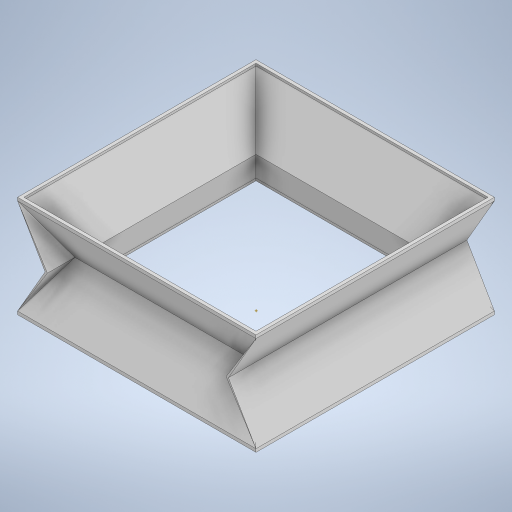
# Autodesk Inventor part: 사각형 OV-PAM 5패턴 층 한개
Saved by Autodesk Inventor 2024 (Build 280153000, 153)
## iProperties
Created: 2023-06-16
Part Number: 사각형 OV-PAM 5패턴 층 한개
Material: 일반
Document SubType Name: Modeling
Designer: jsw
Density: 1 g/cm^3
Appearance: 기본값
Author: jsw
Autodesk Inventor part; units mm, degrees
ref_plane "YZ Plane" through (0, 0, 0) normal (1, 0, 0) x (0, 1, 0)
ref_plane "XZ Plane" through (0, 0, 0) normal (0, 1, 0) x (-1, 0, 0)
ref_plane "XY Plane" through (0, 0, 0) normal (0, 0, 1) x (1, 0, 0)
sketch "스케치1" plane through (0, 0, 0) normal (0, 1, 0) x (-1, 0, 0)
  line L0 (0, 0) -> (-60, 0)
  line L1 (-60, 0) -> (-60, -60)
  line L2 (-60, -60) -> (0, -60)
  line L3 (0, -60) -> (0, 0)
  dimension "d0" = 60
  dimension "d1" = 60
  constraints: 8 end point, 2 parallel, 1 horizontal, 1 perpendicular
  measures "d0" distance of L2.end L1.end
  measures "d1" distance of L1.end L0.end
extrude "돌출1" add sketch "스케치1" along normal blind 12
ref_plane "작업 평면1" through (0, 0, 0) normal (0, 0.5, 0.8660254) x (1, 0, 0)
sketch "스케치2" plane through (0, 0, 0) normal (0, 0, 1) x (1, 0, 0)
  line L0 (60, 0) -> (0, 0) projected
  line L1 (0, 0) -> (7.5, 12)
  line L2 (60, 12) -> (0, 12) projected
  line L3 (60, 0) -> (52.5, 12)
  line L4 (7.5, 12) -> (52.5, 12)
  line L5 (60, 0) -> (0, 0)
  point P0 (52.5, 12)
  point P1 (30, 12)
  dimension "d27" = 45
  dimension "d28" = 22.5
  constraints: 8 end point, 2 collinear, 1 midpoint, 1 point on line
  measures "d27" distance of L1.end L3.end
  measures "d28" distance of L1.end point (30, 12)
extrude "돌출2" cut sketch "스케치2" against normal up to surface surface through (0, 0, 0) normal (0, 0.5, 0.8660254)
ref_plane "작업 평면2" through (60, 0, 0) normal (0.8660254, 0.5, 0) x (0, 0, -1)
sketch "스케치3" plane through (60, 0, -60) normal (1, 0, 0) x (0, 0, -1)
  line L0 (0, 12) -> (-60, 12) projected
  line L1 (-60, 12) -> (0, 12)
  line L2 (0, 12) -> (0, 0)
  line L3 (0, 0) -> (-60, 0)
  line L4 (-60, 0) -> (-60, 12)
  line L5 (-60, 0) -> (-66.9282, 12)
  line L6 (-66.9282, 12) -> (-60, 12)
  line L7 (0, 0) -> (6.9282, 12)
  line L8 (6.9282, 12) -> (0, 12)
  dimension "d11" = 120
  dimension "d12" = 120
  constraints: 16 end point, 2 collinear, 2 parallel, 1 horizontal, 1 perpendicular, 1 point on line
  measures "d11" angle of L5 L3
  measures "d12" angle of L3 L7
extrude "돌출3" cut sketch "스케치3" against normal up to surface surface through (60, 0, 0) normal (0.8660254, 0.5, 0)
pattern_circular "원형 패턴1" count 2 over 360 about axis through (30, 0, -30) along (0, -1, 0) of "돌출3", "돌출2"
mirror "미러1" about plane through (30, 12, -30) normal (0, 1, 0) of "돌출3", "돌출2", "돌출1", "원형 패턴1"
sketch "스케치6" plane through (0, 24, -60) normal (0, 1, 0) x (1, 0, 0)
  line L0 (60, -60) -> (60, 0) projected
  line L1 (60, 0) -> (0, 0) projected
  line L2 (0, 0) -> (0, -60) projected
  line L3 (0, -60) -> (60, -60) projected
extrude "돌출6" add sketch "스케치6" along normal blind 0.8
ref_plane "작업 평면4" through (0, 12, 0) normal (0, -1, 0) x (1, 0, 0)
mirror "미러3" about plane through (0, 12, 0) normal (0, -1, 0) of "돌출6"
shell "쉘4" thickness 0.8 removed faces 2 at (20, 24.8, -40) at (20, -0.8, -40)
equation "\"d28\" = 0.5 * d27"
